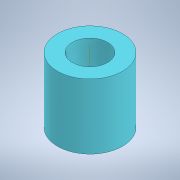
# Autodesk Inventor part: outerShell
Saved by Autodesk Inventor 2021.1 (Build 251245000, 245)
## iProperties
Created: 2020-08-16
Part Number: outerShell
Material: Generic
Document SubType Name: Modeling
Designer: robst
Density: 1 g/cm^3
Appearance: Cadet Blue
Author: robst
Autodesk Inventor part; units mm, degrees
ref_plane "YZ Plane" through (0, 0, 0) normal (1, 0, 0) x (0, 1, 0)
ref_plane "XZ Plane" through (0, 0, 0) normal (0, 1, 0) x (-1, 0, 0)
ref_plane "XY Plane" through (0, 0, 0) normal (0, 0, 1) x (1, 0, 0)
sketch "Sketch1" plane through (0, 0, 0) normal (0, 1, 0) x (-1, 0, 0)
  circle A0 centre (0, 0) radius 38.1
  circle A1 centre (0, 0) radius 20.6375
  dimension "d0" = 76.2
  dimension "d10" = 41.275
  constraints: 2 centre point, 2 coincident
  measures "d0" diameter of A0
  measures "d10" diameter of A1
extrude "Extrusion2" add sketch "Sketch1" along normal blind 76.2
sketch "Sketch6" plane through (0, 0, 0) normal (1, 0, 0) x (0, 1, 0)
  line L0 (76.2, -20.6375) -> (0, -20.6375) projected
  line L1 (76.2, 20.6375) -> (76.2, -20.6375) projected
  line L2 (76.2, -20.6375) -> (82.6905, -31.8794)
  line L3 (82.6905, -31.8794) -> (89.181, -20.6375)
  line L4 (89.181, -20.6375) -> (76.2, -20.6375)
  line L5 (76.2, -38.1) -> (76.2, 38.1) projected
  point P0 (0, 0)
  dimension "d31" = 60
  constraints: 6 end point, 1 collinear, 1 equal length, 1 perpendicular
  measures "d31" angle of L3 L2
body "Solid2"
